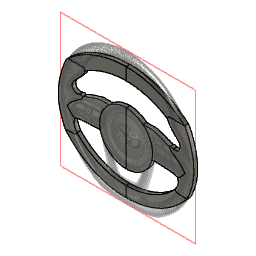
Type 1 v1 (Autodesk Fusion 360 design; units mm, degrees)
Autodesk Fusion 360 part; units mm, degrees
sketch "Centrum" plane through (0, 0, 0) normal (0, 1, 0) x (1, 0, 0)
  circle A0 centre (0, 0) radius 55
  circle A1 centre (0, 0) radius 155
  circle A2 centre (0, 0) radius 197
  constraint coincident A0.centre A1.centre
  constraint concentric A0 A1
sketch "Grip sketch" plane through (0, 0, 0) normal (0, 1, 0) x (1, 0, 0)
  spline S0 degree 5 poles (-161, 59) (-161.5297, 57.9933) (-162.5872, 55.9202) (-164.168, 52.6308) (-166.2646, 47.8842) (-168.8561, 41.3401) (-171.3853, 34.1703) (-173.7873, 26.358) (-175.9506, 17.885) (-177.7311, 8.7418) (-178.9773, -1.0602) (-179.5518, -11.476) (-179.3558, -22.4129) (-178.3507, -33.7173) (-176.59, -45.1541) (-174.2019, -56.4269) (-171.3607, -67.2089) (-168.2632, -77.1696) (-165.104, -86.0045) (-162.053, -93.4616) (-159.2275, -99.3782) (-157.1896, -102.8306) (-155.7936, -104.6957) (-154.9214, -105.6186) (-154.5, -106) knots 0 0 0 0 0 0 0.05 0.1 0.15 0.2 0.25 0.3 0.35 0.4 0.45 0.5 0.55 0.6 0.65 0.7 0.75 0.8 0.85 0.9 0.95 1 1 1 1 1 1
  line L0 (-154.5, -106) -> (-118, -106)
  spline S1 degree 5 poles (-118, -106) (-117.4862, -106.0149) (-116.5002, -106.0165) (-115.1454, -105.9342) (-113.5886, -105.655) (-112.0588, -105.0231) (-110.9405, -104.1122) (-110.2189, -102.9339) (-109.8639, -101.5107) (-109.8388, -99.8726) (-110.1074, -98.0533) (-110.6444, -96.0864) (-111.4361, -94.003) (-112.4739, -91.8321) (-113.7499, -89.6001) (-115.2519, -87.3302) (-116.9569, -85.0425) (-118.8309, -82.7534) (-120.8334, -80.4765) (-122.9205, -78.2225) (-125.0486, -76.0001) (-127.1777, -73.8154) (-129.2749, -71.6729) (-131.3178, -69.5754) (-133.2921, -67.5242) (-135.1898, -65.52) (-136.6439, -63.9542) (-137.6982, -62.8008) (-138.3849, -62.0412) (-138.7242, -61.6638) knots 0 0 0 0 0 0 0.04 0.08 0.12 0.16 0.2 0.24 0.28 0.32 0.36 0.4 0.44 0.48 0.52 0.56 0.6 0.64 0.68 0.72 0.76 0.8 0.84 0.88 0.92 0.96 1 1 1 1 1 1
  spline S2 degree 5 poles (-161, 59) (-160.6117, 59.0309) (-159.8163, 59.0878) (-158.5666, 59.1581) (-156.7863, 59.2216) (-154.3699, 59.2483) (-151.7682, 59.2184) (-149.0004, 59.1253) (-146.1049, 58.9599) (-143.1501, 58.7105) (-140.2358, 58.3629) (-137.4787, 57.9012) (-135.0012, 57.3097) (-132.9178, 56.5737) (-131.3236, 55.6817) (-130.2755, 54.628) (-129.8864, 53.656) (-129.8461, 52.8556) (-129.9302, 52.2904) (-130, 52) knots 0 0 0 0 0 0 0.066667 0.133333 0.2 0.266667 0.333333 0.4 0.466667 0.533333 0.6 0.666667 0.733333 0.8 0.866667 0.933333 1 1 1 1 1 1
  spline S3 degree 5 poles (-130, 52) (-130.22, 51.6667) (-130.6578, 50.9921) (-131.3077, 49.9568) (-132.1605, 48.5288) (-133.2006, 46.6635) (-134.207, 44.7174) (-135.1645, 42.6932) (-136.0484, 40.5982) (-136.8226, 38.4461) (-137.4455, 36.2541) (-137.8742, 34.0406) (-138.0707, 31.8229) (-138.0075, 29.6147) (-137.6738, 27.4246) (-137.0688, 25.2569) (-136.3716, 23.542) (-135.7312, 22.2668) (-135.2524, 21.4214) (-135, 21) knots 0 0 0 0 0 0 0.066667 0.133333 0.2 0.266667 0.333333 0.4 0.466667 0.533333 0.6 0.666667 0.733333 0.8 0.866667 0.933333 1 1 1 1 1 1
  spline S4 degree 5 poles (-135, 21) (-135.129, 21.033) (-135.3924, 21.088) (-135.8038, 21.1373) (-136.3855, 21.1364) (-137.1718, 21.0168) (-138.0279, 20.7618) (-138.9725, 20.3419) (-140.0275, 19.7228) (-141.2145, 18.8713) (-142.5486, 17.7644) (-144.0355, 16.3948) (-145.6747, 14.7649) (-147.4618, 12.8831) (-149.3907, 10.7606) (-151.4549, 8.4089) (-153.2101, 6.3517) (-154.5832, 4.7129) (-155.5236, 3.578) (-156, 3) knots 0 0 0 0 0 0 0.066667 0.133333 0.2 0.266667 0.333333 0.4 0.466667 0.533333 0.6 0.666667 0.733333 0.8 0.866667 0.933333 1 1 1 1 1 1
  spline S5 degree 5 poles (-156, 3) (-155.6818, 2.5702) (-155.0453, 1.7175) (-154.0905, 0.459) (-152.8172, -1.1777) (-151.2236, -3.1549) (-149.6236, -5.0652) (-148.0083, -6.9132) (-146.3628, -8.7071) (-144.664, -10.4605) (-142.8823, -12.1916) (-140.9889, -13.9181) (-138.9629, -15.6533) (-136.798, -17.4014) (-134.5091, -19.1535) (-132.1417, -20.8817) (-129.7663, -22.5441) (-127.4632, -24.0972) (-125.312, -25.5049) (-123.3778, -26.7501) (-121.7002, -27.8435) (-120.2773, -28.8383) (-119.0755, -29.8167) (-118.0473, -30.8685) (-117.1461, -32.0724) (-116.3428, -33.4745) (-115.7668, -34.7719) (-115.3698, -35.8466) (-115.1207, -36.608) (-115, -37) knots 0 0 0 0 0 0 0.04 0.08 0.12 0.16 0.2 0.24 0.28 0.32 0.36 0.4 0.44 0.48 0.52 0.56 0.6 0.64 0.68 0.72 0.76 0.8 0.84 0.88 0.92 0.96 1 1 1 1 1 1
  spline S6 degree 5 poles (-115, -37) (-114.9722, -37.1458) (-114.9354, -37.4259) (-114.9362, -37.8111) (-115.0501, -38.2546) (-115.3828, -38.6901) (-115.9027, -39.0065) (-116.597, -39.2074) (-117.4362, -39.3039) (-118.3796, -39.312) (-119.3811, -39.2498) (-120.3938, -39.1363) (-121.3753, -38.9888) (-122.2928, -38.8212) (-123.1274, -38.6429) (-123.8699, -38.4592) (-124.3882, -38.3102) (-124.7345, -38.1976) (-124.9466, -38.1223) (-125.048, -38.0846) knots 0 0 0 0 0 0 0.066667 0.133333 0.2 0.266667 0.333333 0.4 0.466667 0.533333 0.6 0.666667 0.733333 0.8 0.866667 0.933333 1 1 1 1 1 1
  line L1 (0, -70) -> (0, 70)
  circle A0 centre (0, 0) radius 70
  spline S7 degree 5 poles (-138.7242, -61.6638) (-139.0689, -61.3377) (-139.7247, -60.6663) (-140.6076, -59.6015) (-141.5813, -58.0657) (-142.4504, -55.9537) (-142.9596, -53.6625) (-143.0974, -51.2249) (-142.8578, -48.7056) (-142.243, -46.2039) (-141.2595, -43.8353) (-139.9171, -41.7174) (-138.2277, -39.9552) (-136.2059, -38.6223) (-133.8693, -37.7529) (-131.2341, -37.3576) (-128.8977, -37.4177) (-127.021, -37.6708) (-125.7148, -37.9314) (-125.048, -38.0846) knots 0 0 0 0 0 0 0.066667 0.133333 0.2 0.266667 0.333333 0.4 0.466667 0.533333 0.6 0.666667 0.733333 0.8 0.866667 0.933333 1 1 1 1 1 1
  spline S8 degree 5 poles (-135, 21) (-134.6572, 20.8089) (-133.9159, 20.436) (-132.6367, 19.9046) (-130.5941, 19.2524) (-127.475, 18.5324) (-123.8009, 17.9077) (-119.6188, 17.3742) (-115.0105, 16.9241) (-110.0743, 16.5474) (-104.9148, 16.2334) (-99.6307, 15.9718) (-94.304, 15.7533) (-88.9892, 15.5708) (-83.7207, 15.4189) (-78.517, 15.294) (-74.412, 15.2137) (-71.3666, 15.1642) (-69.351, 15.1358) (-68.3469, 15.1228) knots 0 0 0 0 0 0 0.066667 0.133333 0.2 0.266667 0.333333 0.4 0.466667 0.533333 0.6 0.666667 0.733333 0.8 0.866667 0.933333 1 1 1 1 1 1
  spline S9 degree 5 poles (-115, -37) (-115.1173, -37.1096) (-115.2153, -37.3628) (-114.9522, -37.8444) (-113.7781, -38.6909) (-110.9657, -40.0806) (-106.9292, -41.7641) (-101.931, -43.6616) (-96.3218, -45.666) (-90.4971, -47.6561) (-84.8523, -49.5094) (-79.7385, -51.1152) (-75.4163, -52.3885) (-72.0131, -53.2819) (-69.4647, -53.8036) (-67.4953, -54.0233) (-65.7335, -54.0399) (-63.7944, -53.9578) (-61.3929, -53.8567) (-58.3564, -53.7862) (-54.5887, -53.776) (-50.9582, -53.8268) (-47.8856, -53.8998) (-45.6824, -53.964) (-44.5421, -54) knots 0 0 0 0 0 0 0.05 0.1 0.15 0.2 0.25 0.3 0.35 0.4 0.45 0.5 0.55 0.6 0.65 0.7 0.75 0.8 0.85 0.9 0.95 1 1 1 1 1 1
  point P0 (-179, -25)
  point P1 (-172, 32)
  point P2 (-163, -91)
  point P3 (-111, -104)
  point P4 (-110, -99)
  point P5 (-114.494, -88.5127)
  point P6 (-127, -74)
  point P7 (-147, 59)
  point P8 (-132, 56)
  point P9 (-135, 43)
  point P10 (-138, 32)
  point P11 (-137.1125, 21)
  point P12 (-141, 19)
  point P13 (-147, -8)
  point P14 (-136, -18)
  point P15 (-123, -27)
  point P16 (-118, -31)
  point P17 (-116, -39)
  point P18 (-121.2599, -39)
  point P19 (-143, -52)
  point P20 (-138.7242, -40.5804)
  point P21 (-125.8828, 18.2855)
  point P22 (-100, 16)
  point P23 (-111, -40)
  point P24 (-73, -53)
  point P25 (-65, -54)
  constraint horizontal L0
  constraint vertical L1
  constraint coincident L1.end A0
  constraint coincident L1.start A0
  constraint coincident A0 S8.end
  constraint coincident A0 S9.end
extrude "Extrude1" add sketch "Grip sketch" along normal blind 5 contours S0 L0 S1 S2 S3 S4 S5 S6 S7 S9 makes body 1
extrude "Extrude2" add sketch "Grip sketch" along normal blind 5 separate body contours S4 S5 S6 A0 S8 S9 makes body 2
extrude "Extrude3" add sketch "Grip sketch" along normal blind 5 separate body contours L1 A0 picked at (-17.1722, -15.7975) makes body 3
extrude "Extrude4" add 1 faces at (-17.1722, 0, 15.7975) along direction (0, -1, 0) blind 5 on bodies 3 bodies 3
extrude "Extrude5" add 1 faces at (-96.6647, 0, 6.329) along direction (0, -1, 0) blind 5 on bodies 2 bodies 2
extrude "Extrude6" add 1 faces at (-154.4813, 0, 26.7387) along direction (0, -1, 0) blind 5 on bodies 1 bodies 1
box "BoxPrimitive1" add length 119 width 135 height 10 placed x (0, 0, -1) y (-1, 0, 0) z (0, 1, 0) at (335, 0, 100) separate body makes body 4
move_body "Move1" bodies 4 to x (1, 0, 0) y (0, 1, 0) z (0, 0, 1) at (-200, 0, 0)
move_body "Move2" bodies 4 to x (1, 0, 0) y (0, 1, 0) z (0, 0, 1) at (0, -20, 0)
move_body "Move3" bodies 4 to x (1, 0, 0) y (0, 1, 0) z (0, 0, 1) at (-67.5, 0, 0)
sketch "Top" plane through (0, 0, 0) normal (0, 1, 0) x (1, 0, 0)
  circle A0 centre (0, 70) radius 234.1928
  circle A1 centre (0, 70) radius 201.6457
  line L0 (0, 0) -> (0, -210)
  line L1 (-154.5, -106) -> (-118, -106)
  spline S0 degree 5 poles (-118, -106) (-117.4862, -106.0149) (-116.5002, -106.0165) (-115.1454, -105.9342) (-113.5886, -105.655) (-112.0588, -105.0231) (-110.9405, -104.1122) (-110.2189, -102.9339) (-109.8639, -101.5107) (-109.8388, -99.8726) (-110.1074, -98.0533) (-110.6444, -96.0864) (-111.4361, -94.003) (-112.4739, -91.8321) (-113.7499, -89.6001) (-115.2519, -87.3302) (-116.9569, -85.0425) (-118.8309, -82.7534) (-120.8334, -80.4765) (-122.9205, -78.2225) (-125.0486, -76.0001) (-127.1777, -73.8154) (-129.2749, -71.6729) (-131.3178, -69.5754) (-133.2921, -67.5242) (-135.1898, -65.52) (-136.6439, -63.9542) (-137.6982, -62.8008) (-138.3849, -62.0412) (-138.7242, -61.6638) knots 0 0 0 0 0 0 0.04 0.08 0.12 0.16 0.2 0.24 0.28 0.32 0.36 0.4 0.44 0.48 0.52 0.56 0.6 0.64 0.68 0.72 0.76 0.8 0.84 0.88 0.92 0.96 1 1 1 1 1 1
  point P0 (0, 70)
  point P1 (-154.5, -106)
  point P2 (-110, -99)
  point P3 (-127, -74)
  point P4 (-111, -104)
  point P5 (-114.494, -88.5127)
  point P6 (-110, -99)
  constraint coincident P0 A0.centre
  constraint coincident A0 P1
  constraint concentric A0 A1
  constraint coincident A1 P6
  constraint coincident L0.start origin
  constraint horizontal L1
sketch "Bottom" plane through (0, 0, 0) normal (0, 1, 0) x (1, 0, 0)
  circle A0 centre (0, -70) radius 206.3056
  circle A1 centre (0, -70) radius 178.2807
  line L0 (0, 0) -> (0, 190)
  spline S0 degree 5 poles (-161, 59) (-160.6117, 59.0309) (-159.8163, 59.0878) (-158.5666, 59.1581) (-156.7863, 59.2216) (-154.3699, 59.2483) (-151.7682, 59.2184) (-149.0004, 59.1253) (-146.1049, 58.9599) (-143.1501, 58.7105) (-140.2358, 58.3629) (-137.4787, 57.9012) (-135.0012, 57.3097) (-132.9178, 56.5737) (-131.3236, 55.6817) (-130.2755, 54.628) (-129.8864, 53.656) (-129.8461, 52.8556) (-129.9302, 52.2904) (-130, 52) knots 0 0 0 0 0 0 0.066667 0.133333 0.2 0.266667 0.333333 0.4 0.466667 0.533333 0.6 0.666667 0.733333 0.8 0.866667 0.933333 1 1 1 1 1 1
  point P0 (0, -70)
  point P1 (-161, 59)
  point P2 (-130, 52)
  point P3 (-132, 56)
  point P4 (-147, 59)
  constraint coincident P0 A0.centre
  constraint coincident A0 P1
  constraint concentric A0 A1
  constraint coincident A1 P2
  constraint coincident L0.start origin
extrude "Extrude7" add sketch "Top" along normal blind 5 separate body contours A0 A1 L0 L1 S0 picked at (-74.0129, -140.1665) makes body 5
extrude "Extrude8" add sketch "Bottom" along normal blind 5 separate body contours A0 A1 L0 S0 picked at (-122.7402, 83.5524) makes body 6
extrude "Extrude9" add 2 faces at (-122.7402, 0, -83.5524) (-74.0129, 0, 140.1665) along direction (0, -1, 0) blind 5 on bodies 5 6 bodies 6 5
mirror "Mirror1" about plane through (0, 0, 0) normal (1, 0, 0) of bodies 1 2 3 5 6 makes body 7 at (154.4813, 5, 26.7387) makes body 8 at (96.6647, 5, 6.329) makes body 9 at (21.7204, 5, -8.5246) makes body 10 at (74.0129, 5, 140.1665) makes body 11 at (122.7402, 5, -83.5524)
extrude "Extrude10" cut 1 faces at (22.5, -16.6667, -19) along direction (0, 0, 1) blind 1 on bodies 4 bodies 4
hidden bodies 4
named bodies: "Grip", "PCB", "Top", "Bottom", "Grip (1)", "Top (1)", "Bottom (1)"
